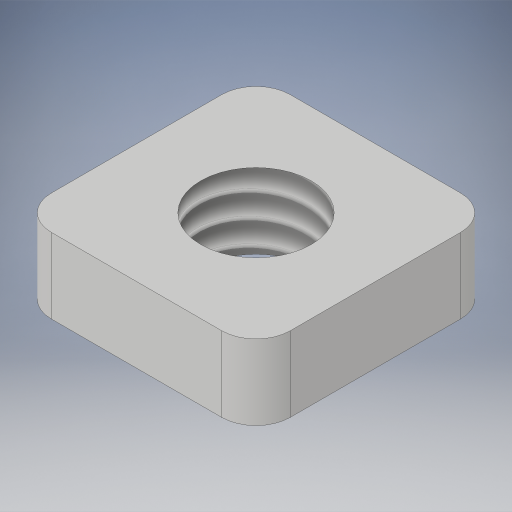
# Autodesk Inventor part: BT004_trajan20_22
Saved by Autodesk Inventor 2023 (Build 270158000, 158)
## iProperties
Company: HTBLA Kaindorf
RuleStatus: InUse
Created: 2022-11-15
Part Number: BT004_trajan20_22
Project: Zeichenmaschine_neu
Material: Generisch
Description: QuadratMutter
Document SubType Name: Modeling
Designer: trajan20
Density: 1 g/cm^3
Appearance: Vorgabe
Mass: 0.0877506 g
Surface Area: 1.60003 cm^2
Volume: 0.0877506 cm^3
AfterDocNew0: iProperties-Editor_aufrufen
Author: jan
Keywords: 2022
Autodesk Inventor part; units mm, degrees
ref_plane "YZ Plane" through (0, 0, 0) normal (1, 0, 0) x (0, 1, 0)
ref_plane "XZ Plane" through (0, 0, 0) normal (0, 1, 0) x (-1, 0, 0)
ref_plane "XY Plane" through (0, 0, 0) normal (0, 0, 1) x (1, 0, 0)
sketch "Skizze3" plane through (0, 0, 0) normal (0, 0, 1) x (1, 0, 0)
  line L0 (0, 0) -> (7, 0)
  line L1 (7, 0) -> (7, 7)
  line L2 (7, 7) -> (0, 7)
  line L3 (0, 7) -> (0, 0)
  point P0 (3.5, 3.5)
  point P1 (3.5, 7)
  point P2 (0, 3.5)
  dimension "d4" = 7
  dimension "d5" = 7
  constraints: 8 end point, 2 midpoint, 2 parallel, 1 horizontal, 1 horizontal alignment, 1 perpendicular, 1 vertical alignment
  measures "d4" distance between parallel lines of L2 L0
  measures "d5" distance between parallel lines of L1 L3
extrude "Extrusion3" add sketch "Skizze3" along normal blind 2.2
fillet "Rundung1" radius 1 4 edges at (7, 7, 1.1) (0, 7, 1.1) (0, 0, 1.1) (7, 0, 1.1)
hole "Bohrung1" at (3.5, 3.5, 0) direction (0, 0, 1) diameter 3.242 depth 11.8 thread size "M4x0.7" class "6H" standard "ISO Metric profile"
equation "\"d5\" = d4"
